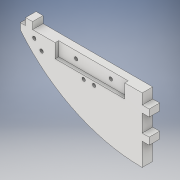
# Autodesk Inventor part: CP004
Saved by Autodesk Inventor 2017 SP1 (Build 210196100, 196)
## iProperties
Created: 2017-05-15
Part Number: CP004
Material: ABS Plastic
Document SubType Name: Modeling
Designer: zallen
Density: 1.06 g/cm^3
Appearance: Smooth - White
Mass: 180.441 g
Surface Area: 330.497 cm^2
Volume: 170.227 cm^3
Author: zallen
Autodesk Inventor part; units mm, degrees
ref_plane "YZ Plane" through (0, 0, 0) normal (1, 0, 0) x (0, 1, 0)
ref_plane "XZ Plane" through (0, 0, 0) normal (0, 1, 0) x (-1, 0, 0)
ref_plane "XY Plane" through (0, 0, 0) normal (0, 0, 1) x (1, 0, 0)
sketch "Sketch1" plane through (0, 0, 0) normal (0, 0, 1) x (1, 0, 0)
  circle A0 centre (0, 132.2876) radius 225 construction
  circle A1 centre (0, 132.2876) radius 200 construction
  line L0 (-225, 132.2876) -> (-150, 132.2876) construction
  line L1 (-150, 132.2876) -> (-150, -35.4175) construction
  line L2 (-175, 132.2876) -> (-175, -9.1338) construction
  line L3 (0, 132.2876) -> (0, -92.7124) construction
  line L4 (-150, 0) -> (0, 0)
  line L5 (-175, -9.1338) -> (-175, 0)
  line L6 (0, 0) -> (0, -92.7124)
  arc A2 (-175, -9.1338) -> (0, -92.7124) centre (0, 132.2876) ccw
  line L7 (-167.5, 0) -> (-167.5, 10)
  line L8 (-167.5, 10) -> (-157.5, 10)
  line L9 (-157.5, 10) -> (-157.5, 0)
  line L10 (-175, 0) -> (-167.5, 0)
  line L11 (-157.5, 0) -> (-150, 0)
  dimension "d0" = 450
  dimension "d1" = 25
  dimension "d2" = 75
  dimension "d3" = 25
  dimension "d14" = 10
  dimension "d15" = 10
  dimension "d16" = 90
  dimension "d17" = 7.5
  constraints: 24 end point, 6 point on circle, 5 point on line, 4 perpendicular, 2 centre point, 2 collinear, 2 horizontal, 2 vertical, 1 coincident, 1 concentric, 3 other
  measures "d0" diameter of A0
  measures "d2" distance of L0.start L0.end
  measures "d3" distance between parallel lines of L1 L2
  measures "d14" distance of L7.start L7.end
  measures "d15" distance of L7.end L8.end
  measures "d16" angle of L7 L8
  measures "d17" distance between parallel lines of L2 L7
extrude "Extrusion1" add sketch "Sketch1" along normal blind 15
sketch "Sketch2" plane through (0, 0, 15) normal (0, 0, 1) x (1, 0, 0)
  line L0 (10, -15) -> (0, -15)
  line L1 (0, -15) -> (0, -25)
  line L2 (0, -25) -> (10, -25)
  line L3 (10, -25) -> (10, -15)
  line L4 (10, -50) -> (0, -50)
  line L5 (0, -50) -> (0, -60)
  line L6 (0, -60) -> (10, -60)
  line L7 (10, -60) -> (10, -50)
  line L8 (0, 0) -> (0, -95.6231) construction
  line L9 (0, -92.7124) -> (0, 0) construction
  dimension "d6" = 10
  dimension "d7" = 10
  dimension "d8" = 10
  dimension "d9" = 10
  dimension "d10" = 15
  dimension "d11" = 25
  constraints: 18 end point, 4 parallel, 2 perpendicular, 2 point on line, 1 collinear
  measures "d6" distance of L2.end L1.end
  measures "d7" distance of L1.end L0.end
  measures "d8" distance of L6.end L5.end
  measures "d9" distance of L5.end L4.end
  measures "d10" distance from line of L8.start L0
  measures "d11" distance between parallel lines of L2 L4
extrude "Extrusion2" add sketch "Sketch2" against normal blind 15
sketch "Sketch3" plane through (0, 0, 15) normal (0, 0, 1) x (1, 0, 0)
  line L0 (-25, 0) -> (-125, 0) construction
  line L1 (-125, 0) -> (-125, -20) construction
  line L2 (-125, -20) -> (-25, -20) construction
  line L3 (-25, -20) -> (-25, 0) construction
  line L4 (0, 0) -> (-157.5, 0) construction
  circle A0 centre (-100, -10) radius 2.5
  circle A1 centre (-50, -10) radius 2.5
  dimension "d18" = 100
  dimension "d19" = 20
  dimension "d20" = 25
  dimension "d21" = 5
  dimension "d22" = 5
  dimension "d23" = 25
  dimension "d24" = 25
  constraints: 8 end point, 2 centre point, 2 parallel, 1 horizontal, 1 perpendicular, 1 point on line
  measures "d18" distance of L2.end L1.end
  measures "d19" distance of L1.end L0.end
  measures "d20" distance from line of L4.start L3
  measures "d21" diameter of A0
  measures "d22" diameter of A1
  measures "d23" distance from line of L1 A0.centre
  measures "d24" distance from line of L3 A1.centre
extrude "Extrusion3" cut sketch "Sketch3" against normal through all
thread "Thread1" size "M5x0.8" class "6H" standard "ANSI Metric M Profile" full length
thread "Thread2" size "M5x0.8" class "6H" standard "ANSI Metric M Profile" full length
sketch "Sketch5" plane through (0, 0, 15) normal (0, 0, 1) x (1, 0, 0)
  line L0 (-125, 0) -> (-25, 0)
  line L1 (-25, 0) -> (-25, -20)
  line L2 (-25, -20) -> (-125, -20)
  line L3 (-125, -20) -> (-125, 0)
  point P0 (0, 0)
  dimension "d31" = 100
  dimension "d32" = 20
  dimension "d33" = 25
  constraints: 8 end point, 2 parallel, 1 horizontal, 1 perpendicular
  measures "d31" distance of L1.end L2.end
  measures "d32" distance of L0.end L1.end
  measures "d33" distance from line of point (0, 0) L1
extrude "Extrusion4" cut sketch "Sketch5" against normal blind 5
sketch "Sketch6" plane through (0, 0, 15) normal (0, 0, 1) x (1, 0, 0)
  circle A0 centre (0, 132.2876) radius 225 construction
  arc A1 (-175, -9.1338) -> (0, -92.7124) centre (0, 132.2876) ccw construction
  circle A2 centre (0, 132.2876) radius 210 construction
  circle A3 centre (-155, -9.3987) radius 2.5
  circle A4 centre (-144.4906, -20.1016) radius 2.5
  line L0 (-175, 0) -> (-175, -9.1338) projected
  point P0 (0, 0)
  dimension "d36" = 450
  dimension "d37" = 15
  dimension "d38" = 5
  dimension "d39" = 5
  dimension "d40" = 15
  dimension "d41" = 20
  constraints: 4 centre point, 2 point on circle, 1 concentric
  measures "d36" diameter of A0
  measures "d37" radial gap between concentric circles of A0 A2
  measures "d38" diameter of A3
  measures "d39" diameter of A4
  measures "d40" distance of A4.centre A3.centre
  measures "d41" distance from line of A3.centre L0
extrude "Extrusion5" cut sketch "Sketch6" against normal through all
thread "Thread3" size "M5x0.8" class "6H" standard "ANSI Metric M Profile" full length
thread "Thread4" size "M5x0.8" class "6H" standard "ANSI Metric M Profile" full length
sketch "Sketch7" plane through (0, 0, 15) normal (0, 0, 1) x (1, 0, 0)
  circle A0 centre (-84.0912, -25.1338) radius 2.5
  circle A1 centre (-69.0912, -25.1338) radius 2.5
  line L0 (-125, 0) -> (-25, 0) projected
  line L1 (-175, 0) -> (-175, -9.1338) construction
  line L2 (-175, -9.1338) -> (22.4277, -9.1338) construction
  point P0 (0, 0)
  dimension "d48" = 5
  dimension "d49" = 5
  dimension "d50" = 69.0912
  dimension "d51" = 15
  dimension "d53" = 16
  constraints: 2 centre point, 2 end point, 1 horizontal
  measures "d48" diameter of A0
  measures "d49" diameter of A1
  measures "d50" horizontal distance of point (0, 0) A1.centre
  measures "d51" distance of A0.centre A1.centre
  measures "d53" distance from line of L2 A1.centre
extrude "Extrusion6" cut sketch "Sketch7" against normal through all
thread "Thread5" size "M5x0.8" class "6H" standard "ANSI Metric M Profile" full length
thread "Thread6" size "M5x0.8" class "6H" standard "ANSI Metric M Profile" full length
body "Solid1"
